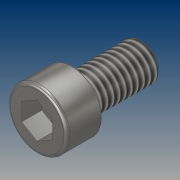
# Autodesk Inventor part: fillament guide screw
Saved by Autodesk Inventor 2019 (Build 230136000, 136)
## iProperties
Created: 2018-11-18
Part Number: fillament guide screw
Material: Steel, Alloy
Document SubType Name: Modeling
Designer: LillaHunden
Density: 7.73 g/cm^3
Appearance: Semi-Polished
Author: LillaHunden
Autodesk Inventor part; units mm, degrees
ref_plane "YZ Plane" through (0, 0, 0) normal (1, 0, 0) x (0, 1, 0)
ref_plane "XZ Plane" through (0, 0, 0) normal (0, 1, 0) x (-1, 0, 0)
ref_plane "XY Plane" through (0, 0, 0) normal (0, 0, 1) x (1, 0, 0)
sketch "Sketch1" plane through (0, 0, 0) normal (0, 0, 1) x (1, 0, 0)
  circle A0 centre (0, 0) radius 3
  dimension "d0" = 6
  constraints: 1 centre point, 1 coincident
  measures "d0" diameter of A0
extrude "Extrusion1" add sketch "Sketch1" along normal blind 11.5
sketch "Sketch2" plane through (0, 0, 11.5) normal (0, 0, 1) x (1, 0, 0)
  circle A0 centre (0, 0) radius 4.875
  dimension "d3" = 9.75
  constraints: 1 centre point, 1 coincident
  measures "d3" diameter of A0
extrude "Extrusion2" add sketch "Sketch2" along normal blind 5.8
sketch "Sketch3" plane through (0, 0, 17.3) normal (0, 0, 1) x (1, 0, 0)
  line L0 (2.5331, -1.4625) -> (0, -2.925)
  line L1 (0, -2.925) -> (-2.5331, -1.4625)
  line L2 (-2.5331, -1.4625) -> (-2.5331, 1.4625)
  line L3 (-2.5331, 1.4625) -> (0, 2.925)
  line L4 (0, 2.925) -> (2.5331, 1.4625)
  line L5 (2.5331, 1.4625) -> (2.5331, -1.4625)
  point P0 (0, 0)
  point P1 (0, 0)
  point P2 (2.5331, 0)
  dimension "d6" = 5.85
  constraints: 12 end point, 1 coincident, 1 horizontal alignment, 1 midpoint, 13 other
  measures "d6" distance of L0.end L3.end
extrude "Extrusion3" cut sketch "Sketch3" against normal blind 3.3
sketch "Sketch4" plane through (0, 0, 14) normal (0, 0, 1) x (1, 0, 0)
  circle A0 centre (0, 0) radius 1
  dimension "d9" = 2
  constraints: 1 centre point, 1 coincident
  measures "d9" diameter of A0
extrude "Extrusion4" cut sketch "Sketch4" against normal through all
chamfer "Chamfer1" distance 0.5 angle 45 1 edges at (-1, 0, 14)
fillet "Fillet1" radius 0.5 1 edges at (-4.875, 0, 17.3)
fillet "Fillet2" radius 0.2 1 edges at (-4.875, 0, 11.5)
thread "Thread1" size "M6x1" class "6g" standard "ISO Metric profile" full length
chamfer "Chamfer2" distance 0.5 angle 45 1 edges at (-3, 0, 0)
body "Solid1"
